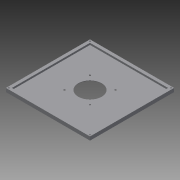
# Autodesk Inventor part: brain box top
Saved by Autodesk Inventor 2015 (Build 190159000, 159)
## iProperties
Created: 2014-10-23
Part Number: brain box top
Material: Generic
Document SubType Name: Modeling
Designer: ericd_000
Density: 1 g/cm^3
Appearance: Default
Author: ericd_000
Autodesk Inventor part; units mm, degrees
ref_plane "YZ Plane" through (0, 0, 0) normal (1, 0, 0) x (0, 1, 0)
ref_plane "XZ Plane" through (0, 0, 0) normal (0, 1, 0) x (-1, 0, 0)
ref_plane "XY Plane" through (0, 0, 0) normal (0, 0, 1) x (1, 0, 0)
sketch "Sketch1" plane through (0, 0, 0) normal (0, 0, 1) x (1, 0, 0)
  line L0 (-140, 140) -> (140, 140)
  line L1 (140, 140) -> (140, -140)
  line L2 (140, -140) -> (-140, -140)
  line L3 (-140, -140) -> (-140, 140)
  point P0 (0, 0)
  point P1 (0, 140)
  point P2 (140, 0)
  dimension "d0" = 280
  dimension "d1" = 280
  constraints: 8 end point, 2 midpoint, 2 parallel, 1 horizontal, 1 horizontal alignment, 1 perpendicular, 1 vertical alignment
  measures "d0" distance of L0.start L0.end
  measures "d1" distance of L2.end L0.start
extrude "Extrusion1" add sketch "Sketch1" along normal blind 6
sketch "Sketch2" plane through (0, 0, 6) normal (0, 0, 1) x (1, 0, 0)
  line L0 (140, 140) -> (-140, 140)
  line L1 (-140, 140) -> (-140, -140)
  line L2 (-140, -140) -> (140, -140)
  line L3 (140, -140) -> (140, 140)
  line L4 (130, 130) -> (-130, 130)
  line L5 (-130, 130) -> (-130, -130)
  line L6 (-130, -130) -> (130, -130)
  line L7 (130, -130) -> (130, 130)
  point P0 (0, 0)
  dimension "d4" = 10
  constraints: 16 end point, 4 parallel, 2 perpendicular, 1 horizontal, 3 other
  measures "d4" distance between parallel lines of L3 L7
extrude "Extrusion2" add sketch "Sketch2" along normal blind 6
sketch "Sketch3" plane through (0, 0, 12) normal (0, 0, 1) x (1, 0, 0)
  circle A0 centre (-135, -135) radius 2.05
  circle A1 centre (-135, 135) radius 2.05
  line L0 (-135, 135) -> (-135, -135) construction
  line L1 (-140, 140) -> (-140, -140) construction
  line L2 (-140, -140) -> (140, -140) construction
  point P0 (0, 0)
  point P1 (-135, 0)
  point P2 (-140, 0)
  dimension "d7" = 4.1
  dimension "d8" = 4.1
  dimension "d9" = 5
  dimension "d10" = 5
  constraints: 2 centre point, 2 end point, 2 midpoint, 1 horizontal alignment, 1 parallel
  measures "d7" diameter of A0
  measures "d8" diameter of A1
  measures "d9" distance between parallel lines of L1 L0
  measures "d10" distance from line of L2 L0.end
extrude "Extrusion3" cut sketch "Sketch3" against normal up to surface (12 mm away)
mirror "Mirror1" about plane through (0, 0, 0) normal (1, 0, 0) of "Extrusion3"
sketch "Sketch4" plane through (0, 0, 0) normal (0, 0, -1) x (-1, 0, 0)
  line L0 (-52.5, 52.5) -> (52.5, 52.5)
  line L1 (52.5, 52.5) -> (52.5, -52.5)
  line L2 (52.5, -52.5) -> (-52.5, -52.5)
  line L3 (-52.5, -52.5) -> (-52.5, 52.5)
  point P0 (0, 0)
  point P1 (52.5, 0)
  point P2 (0, 52.5)
  dimension "d13" = 105
  dimension "d14" = 105
  constraints: 8 end point, 2 midpoint, 2 parallel, 1 horizontal, 1 horizontal alignment, 1 perpendicular, 1 vertical alignment
  measures "d13" distance of L0.start L0.end
  measures "d14" distance of L0.end L1.end
extrude "Extrusion4" cut sketch "Sketch4" against normal blind 5
sketch "Sketch5" plane through (0, 0, 5) normal (0, 0, -1) x (-1, 0, 0)
  circle A0 centre (0, 0) radius 39
  dimension "d17" = 78
  constraints: 1 centre point, 1 coincident
  measures "d17" diameter of A0
extrude "Extrusion5" cut sketch "Sketch5" against normal blind 5
sketch "Sketch6" plane through (0, 0, 5) normal (0, 0, -1) x (-1, 0, 0)
  circle A0 centre (-42.5, 42.5) radius 2.75
  line L0 (-52.5, 52.5) -> (52.5, 52.5) projected
  line L1 (-52.5, -52.5) -> (-52.5, 52.5) projected
  point P0 (0, 0)
  dimension "d27" = 5.5
  dimension "d28" = 10
  dimension "d29" = 10
  constraints: 1 centre point
  measures "d27" diameter of A0
  measures "d28" distance from line of A0.centre L0
  measures "d29" distance from line of L1 A0.centre
extrude "Extrusion6" cut sketch "Sketch6" against normal blind 5
pattern_linear "Rectangular Pattern1" count 2 spacing 85 along (0, -1, 0) count 2 spacing 85 along (-1, 0, 0) of "Extrusion6"
body "Solid1"
